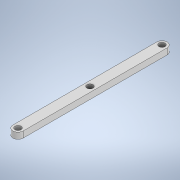
# Autodesk Inventor part: tussenarm
Saved by Autodesk Inventor 2022 (Build 260153000, 153)
## iProperties
Created: 2021-12-23
Part Number: tussenarm
Material: Generic
Document SubType Name: Modeling
Designer: keemi
Density: 1 g/cm^3
Appearance: Default
Author: keemi
Autodesk Inventor part; units mm, degrees
ref_plane "YZ Plane" through (0, 0, 0) normal (1, 0, 0) x (0, 1, 0)
ref_plane "XZ Plane" through (0, 0, 0) normal (0, 1, 0) x (-1, 0, 0)
ref_plane "XY Plane" through (0, 0, 0) normal (0, 0, 1) x (1, 0, 0)
sketch "Sketch1" plane through (0, 0, 0) normal (0, 1, 0) x (-1, 0, 0)
  line L0 (0, 0) -> (0, -35)
  line L1 (0, -35) -> (0, -70)
  circle A0 centre (0, 0) radius 2.5
  circle A1 centre (0, -70) radius 2.5
  circle A2 centre (0, 0) radius 1.5
  circle A3 centre (0, -35) radius 1.5
  circle A4 centre (0, -70) radius 1.5
  line L2 (2.5, 0) -> (2.5, -70)
  line L3 (-2.5, 0) -> (-2.5, -70)
  dimension "d0" = 35
  dimension "d1" = 35
  dimension "d2" = 5
  dimension "d3" = 5
  dimension "d4" = 3
  dimension "d5" = 3
  dimension "d6" = 3
  constraints: 8 end point, 5 centre point, 5 coincident, 4 point on circle, 2 tangent, 1 point on line, 1 vertical
  measures "d0" distance of L0.start L0.end
  measures "d1" distance of L0.end L1.end
  measures "d2" diameter of A0
  measures "d3" diameter of A1
  measures "d4" diameter of A2
  measures "d5" diameter of A3
  measures "d6" diameter of A4
extrude "Extrusion1" add sketch "Sketch1" along normal blind 3 contours A0 | A0 L2 A1 L1 A3 L0 | L0 A3 L1 A1 L3 A0 | A1
body "Solid1"
